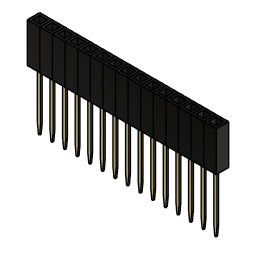
female_header_pins (Autodesk Fusion 360 design; units mm, degrees)
part number: 2025-05-23-10-09-07-370
Autodesk Fusion 360 part; units mm, degrees
sketch "Plastic casing" plane through (0, 0, 0) normal (0, 1, 0) x (1, 0, 0)
  line L0 (0, 0) -> (2.54, 0)
  line L1 (2.54, 0) -> (2.54, -8)
  line L2 (2.54, -8) -> (0, -8)
  line L3 (0, -8) -> (0, 0)
  dimension "d1" = 8
  dimension "d2" = 2.54
  constraint horizontal L0
  constraint vertical L1
  constraint horizontal L2
  constraint vertical L3
  constraint coincident L0.start L3.end
  measures "d1" distance of L0.end L1.end
  measures "d2" distance of L0.start L0.end
extrude "Extrude1" add sketch "Plastic casing" along normal blind 2.5 makes body 1
sketch "Hole" plane through (0, 0, 8) normal (0, 0, 1) x (-1, 0, 0)
  line L0 (0, 0) -> (-2.54, 0)
  line L1 (-2.54, 0) -> (-2.54, -2.5)
  line L2 (-2.54, -2.5) -> (0, -2.5)
  line L3 (0, -2.5) -> (0, 0)
  line L4 (-0.5, -2) -> (-2.04, -2)
  line L5 (-2.04, -2) -> (-2.04, -0.5)
  line L6 (-2.04, -0.5) -> (-0.5, -0.5)
  line L7 (-0.5, -0.5) -> (-0.5, -2)
  dimension "d6" = 0.5
  dimension "d7" = 0.5
  dimension "d8" = 0.5
  dimension "d9" = 0.5
  constraint horizontal L4
  constraint vertical L5
  constraint horizontal L6
  constraint vertical L7
  measures "d6" distance of L2 L4
  measures "d7" distance of L0 L6
  measures "d8" distance of L3 L7
  measures "d9" distance of L1 L5
extrude "Extrude2" cut sketch "Hole" against normal blind 7 contours L4 L5 L6 L7 bodies 1
sketch "Pin" plane through (0, 0, 0) normal (0, 0, 1) x (1, 0, 0)
  line L0 (2.54, 0) -> (0, 0)
  line L1 (0, 0) -> (0, 2.5)
  line L2 (0, 2.5) -> (2.54, 2.5)
  line L3 (2.54, 2.5) -> (2.54, 0)
  line L4 (0.945, 1.09) -> (1.595, 1.09)
  line L5 (1.595, 1.09) -> (1.595, 1.41)
  line L6 (1.595, 1.41) -> (0.945, 1.41)
  line L7 (0.945, 1.41) -> (0.945, 1.09)
  dimension "d12" = 0.65
  dimension "d13" = 0.32
  dimension "d14" = 0.945
  dimension "d15" = 0.945
  dimension "d16" = 1.09
  dimension "d17" = 1.09
  constraint horizontal L4
  constraint vertical L5
  constraint horizontal L6
  constraint vertical L7
  measures "d12" distance of L5.end L6.end
  measures "d13" distance of L4.end L5.end
  measures "d14" distance of L1 L7
  measures "d15" distance of L3 L5
  measures "d16" distance of L2 L6
  measures "d17" distance of L0 L4
extrude "Extrude3" add sketch "Pin" against normal blind 12 separate body contours L4 L5 L6 L7 makes body 2
chamfer "Chamfer1" distance 0.2 distance2 2 2 edges at (1.595, 1.25, -12) (0.945, 1.25, -12) measured on face at (1.1617, 1.3033, -12) measured on face at (1.1617, 1.3033, -12) on bodies 2
pattern_linear "R-Pattern1" count 15 spacing 2.54 along (1, 0, 0) of bodies 1 2 makes body 3 at (3.3867, 0, 2.6667) makes body 4 at (5.9267, 0, 2.6667) makes body 5 at (8.4667, 0, 2.6667) makes body 6 at (11.0067, 0, 2.6667) makes body 7 at (13.5467, 0, 2.6667) makes body 8 at (16.0867, 0, 2.6667) makes body 9 at (18.6267, 0, 2.6667) makes body 10 at (21.1667, 0, 2.6667) makes body 11 at (23.7067, 0, 2.6667) makes body 12 at (26.2467, 0, 2.6667) makes body 13 at (28.7867, 0, 2.6667) makes body 14 at (31.3267, 0, 2.6667) makes body 15 at (33.8667, 0, 2.6667) makes body 16 at (36.4067, 0, 2.6667) makes body 17 at (3.9183, 1.41, -3.3333) makes body 18 at (6.4583, 1.41, -3.3333) makes body 19 at (8.9983, 1.41, -3.3333) makes body 20 at (11.5383, 1.41, -3.3333) makes body 21 at (14.0783, 1.41, -3.3333) makes body 22 at (16.6183, 1.41, -3.3333) makes body 23 at (19.1583, 1.41, -3.3333) makes body 24 at (21.6983, 1.41, -3.3333) makes body 25 at (24.2383, 1.41, -3.3333) makes body 26 at (26.7783, 1.41, -3.3333) makes body 27 at (29.3183, 1.41, -3.3333) makes body 28 at (31.6417, 1.09, -3.3333) makes body 29 at (34.3983, 1.41, -3.3333) makes body 30 at (36.9383, 1.41, -3.3333)
equation "d14 = ( ( 2.54 - 0.65 ) / 2 ) * 1 mm"
equation "d16 = ( ( 2.5 - 0.32 ) / 2 ) * 1 mm"
named bodies: "Plastic Casing", "Pin", "Plastic Casing (1)", "Plastic Casing (2)", "Plastic Casing (3)", "Plastic Casing (4)", "Plastic Casing (5)", "Plastic Casing (6)", "Plastic Casing (7)", "Plastic Casing (8)", "Plastic Casing (9)", "Plastic Casing (10)", "Plastic Casing (11)", "Plastic Casing (12)", "Plastic Casing (13)", "Plastic Casing (14)", "Pin (1)", "Pin (2)", "Pin (3)", "Pin (4)", "Pin (5)", "Pin (6)", "Pin (7)", "Pin (8)", "Pin (9)", "Pin (10)", "Pin (11)", "Pin (12)", "Pin (13)", "Pin (14)"
